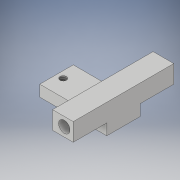
# Autodesk Inventor part: slide to axle bracet
Saved by Autodesk Inventor 2019 (Build 230136000, 136)
## iProperties
Created: 2018-12-13
Part Number: slide to axle bracet
Material: Generic
Document SubType Name: Modeling
Designer: User
Density: 1 g/cm^3
Appearance: Default
Author: User
Autodesk Inventor part; units mm, degrees
ref_plane "YZ Plane" through (0, 0, 0) normal (1, 0, 0) x (0, 1, 0)
ref_plane "XZ Plane" through (0, 0, 0) normal (0, 1, 0) x (-1, 0, 0)
ref_plane "XY Plane" through (0, 0, 0) normal (0, 0, 1) x (1, 0, 0)
sketch "Sketch1" plane through (0, 0, 0) normal (0, 1, 0) x (-1, 0, 0)
  line L0 (0, 0) -> (38.1, 0)
  line L1 (38.1, 0) -> (38.1, -19.05)
  line L2 (38.1, -19.05) -> (0, -19.05)
  line L3 (0, -19.05) -> (0, 0)
  dimension "d0" = 38.1
  dimension "d1" = 19.05
  constraints: 8 end point, 2 parallel, 1 horizontal, 1 perpendicular
  measures "d0" distance of L1.end L2.end
  measures "d1" distance of L0.end L1.end
extrude "Extrusion1" add sketch "Sketch1" along normal blind 6.35
sketch "Sketch2" plane through (0, 6.35, 0) normal (0, 1, 0) x (1, 0, 0)
  line L0 (0, 19.05) -> (-38.1, 19.05) projected
  line L1 (0, -19.05) -> (-11.7718, -19.05)
  line L2 (-11.7718, -19.05) -> (-11.7718, 38.1)
  line L3 (-11.7718, 38.1) -> (0, 38.1)
  line L4 (0, 38.1) -> (0, -19.05)
  line L5 (-38.1, 0) -> (0, 0) projected
  dimension "d22" = 19.05
  dimension "d38" = 19.05
  constraints: 8 end point, 2 parallel, 1 horizontal, 1 perpendicular
  measures "d22" distance between parallel lines of L3 L0
  measures "d38" distance between parallel lines of L5 L1
extrude "Extrusion2" add sketch "Sketch2" along normal blind 10.16
sketch "Sketch3" plane through (-38.1, 0, 0) normal (0, 0, 1) x (1, 0, 0)
  line L0 (38.1, 0) -> (0, 0) projected
  line L1 (38.1, 0) -> (38.1, 6.35) projected
  line L2 (0, 6.35) -> (26.3282, 6.35) projected
  line L3 (0, 0) -> (0, 6.35) projected
  line L4 (26.3282, 6.35) -> (38.1, 6.35) projected
  point P0 (33.02, 11.43)
  dimension "d9" = 5.08
  measures "d9" distance from line of L1 point (33.02, 11.43)
hole "Hole1" at (-5.08, 11.43, 0) direction (0, 0, -1) diameter 6.477 end through all both
sketch "Sketch4" plane through (0, 0, 0) normal (0, -1, 0) x (1, 0, 0)
  line L0 (0, 0) -> (-38.1, 0) projected
  line L1 (-38.1, 0) -> (-38.1, -19.05) projected
  line L2 (-38.1, -19.05) -> (0, -19.05) projected
  line L3 (0, -19.05) -> (0, 0) projected
  point P0 (-34.29, -9.525)
  point P1 (-3.81, -9.525)
  dimension "d23" = 19.05
  dimension "d24" = 38.1
  dimension "d25" = 9.525
  dimension "d26" = 9.525
  dimension "d27" = 3.81
  dimension "d35" = 3.81
  measures "d23" distance of L2.end L0.start
  measures "d24" distance of L0.start L0.end
  measures "d25" distance from line of point (-3.81, -9.525) L0
  measures "d26" distance from line of L0 point (-34.29, -9.525)
  measures "d27" distance from line of L1 point (-34.29, -9.525)
  measures "d35" distance from line of L3 point (-3.81, -9.525)
hole "Hole2" at (-34.29, 0, -9.525) at (-3.81, 0, -9.525) direction (0, 1, 0) diameter 3.683 depth 6.35 tip angle 118 thread size "10-24 UNC" class "2B" standard "ANSI Unified Screw Threads"
fillet "Fillet2" radius 3.175 1 edges at (-11.7718, 6.35, -9.525)
equation "\"d22\" = d38"
equation "\"d9\" = 0.5 * d7"
equation "\"d25\" = 0.5 * d23"
equation "\"d26\" = 0.5 * d23"
equation "\"d7\" = 10.16"
body "Solid1"
